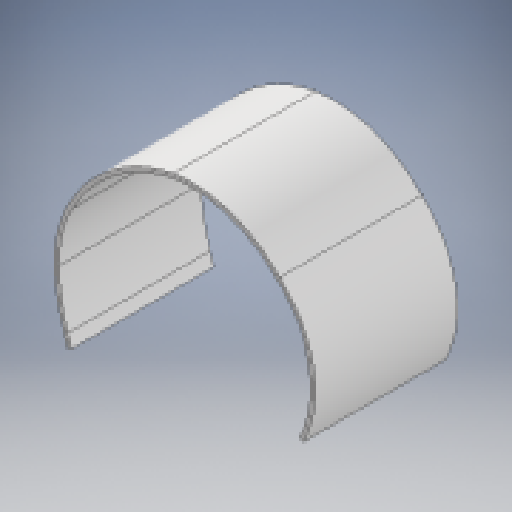
# Autodesk Inventor part: mount3
Saved by Autodesk Inventor 2025.2 (Build 292293000, 293)
## iProperties
Created: 2025-02-11
Part Number: mount3
Material: Generic
Document SubType Name: Modeling
Designer: Alex
Density: 1 g/cm^3
Appearance: Default
Author: Alex
Autodesk Inventor part; units mm, degrees
ref_plane "YZ Plane" through (0, 0, 0) normal (1, 0, 0) x (0, 1, 0)
ref_plane "XZ Plane" through (0, 0, 0) normal (0, 1, 0) x (-1, 0, 0)
ref_plane "XY Plane" through (0, 0, 0) normal (0, 0, 1) x (1, 0, 0)
sketch "Sketch1" plane through (0, 0, 0) normal (0, 0, 1) x (1, 0, 0)
  spline S0 degree 4 poles (-146.6472, 58.0401) (-151.4631, 48.7396) (-154.252, 35.0489) (-156.3713, 15.6625) (-155.4501, -11.3591) (-147.1073, -27.1547) (-140.0741, -39.9858) (-129.6609, -50.3249) (-121.6575, -59.5045) (-108.3024, -68.785) (-98.2709, -73.1981) (-84.1702, -79.7266) (-75.9561, -81.5933) (-64.5094, -82.4436) (-52.8851, -81.3854) (-36.0893, -77.2113) (-27.9896, -73.4594) (-12.8633, -65.2256) (-3.7509, -56.3713) (7.8984, -44.4028) (15.2147, -32.4708) (21.1011, -10.2225) (21.2051, 16.649) (15.9713, 25.1459) (12.5155, 32.2876) knots 0 0 0 0 0 0.111891 0.158364 0.204234 0.248308 0.289897 0.330614 0.370754 0.411053 0.44968 0.486304 0.522824 0.560101 0.5983 0.638491 0.679191 0.71966 0.761289 0.803726 0.849038 0.894451 1 1 1 1 1 construction
  arc A0 (-146.6314, -27.8645) -> (-75.5, -81.3478) centre (-54.4542, 20.6856) ccw construction
  arc A1 (-75.5, -81.3478) -> (-3.571, -56.0466) centre (-63.9052, 0.5835) ccw construction
  arc A2 (-155.7423, 8.5009) -> (-146.6314, -27.8645) centre (-64.0155, 12.158) ccw construction
  arc A3 (-146.6472, 58.0401) -> (-155.7423, 8.5009) centre (-41.1628, 13.0692) ccw construction
  arc A4 (-3.571, -56.0466) -> (18.787, -15.947) centre (-44.8542, -6.7459) ccw construction
  arc A5 (18.787, -15.947) -> (12.5155, 32.2876) centre (-51.5039, -0.5612) ccw construction
  arc A6 (-149.4068, 59.2166) -> (-149.2857, -29.2626) centre (-45.9699, 15.1186) ccw construction
  arc A7 (-149.2857, -29.2626) -> (-75.9204, -84.3182) centre (-62.5938, 9.8502) ccw construction
  arc A8 (-75.9204, -84.3182) -> (-1.3836, -58.0997) centre (-63.9052, 0.5835) ccw construction
  arc A9 (-1.3836, -58.0997) -> (15.1847, 33.6571) centre (-53.1101, -1.3853) ccw construction
  line L0 (-146.6472, 58.0401) -> (-149.4068, 59.2166) construction
  line L1 (-146.6314, -27.8645) -> (-149.2857, -29.2626) construction
  line L2 (-75.5, -81.3478) -> (-75.9204, -84.3182) construction
  line L3 (12.5155, 32.2876) -> (15.1847, 33.6571) construction
  line L4 (-3.571, -56.0466) -> (-1.3836, -58.0997) construction
  line L5 (-266.975, 160) -> (333.025, 160) construction
  line L6 (0, 160) -> (0, 0) construction
  arc A10 (-155.7423, 311.4991) -> (-146.6472, 261.9599) centre (-41.1628, 306.9308) ccw construction
  line L7 (-146.6472, 261.9599) -> (-149.4068, 260.7834) construction
  arc A11 (-149.2857, 349.2626) -> (-149.4068, 260.7834) centre (-45.9699, 304.8814) ccw construction
  spline S1 degree 4 poles (-146.6472, 261.9599) (-151.4631, 271.2604) (-154.252, 284.9511) (-156.3713, 304.3375) (-155.4501, 331.3591) (-147.1073, 347.1547) (-140.0741, 359.9858) (-129.6609, 370.3249) (-121.6575, 379.5045) (-108.3024, 388.785) (-98.2709, 393.1981) (-84.1702, 399.7266) (-75.9561, 401.5933) (-64.5094, 402.4436) (-52.8851, 401.3854) (-36.0893, 397.2113) (-27.9896, 393.4594) (-12.8633, 385.2256) (-3.7509, 376.3713) (7.8984, 364.4028) (15.2147, 352.4708) (21.1011, 330.2225) (21.2051, 303.351) (15.9713, 294.8541) (12.5155, 287.7124) knots 0 0 0 0 0 0.111891 0.158364 0.204234 0.248308 0.289897 0.330614 0.370754 0.411053 0.44968 0.486304 0.522824 0.560101 0.5983 0.638491 0.679191 0.71966 0.761289 0.803726 0.849038 0.894451 1 1 1 1 1 construction
  line L8 (-146.6314, 347.8645) -> (-149.2857, 349.2626) construction
  arc A12 (-75.5, 401.3478) -> (-146.6314, 347.8645) centre (-54.4542, 299.3144) ccw
  arc A13 (-75.9204, 404.3182) -> (-149.2857, 349.2626) centre (-62.5938, 310.1498) ccw construction
  line L9 (-3.571, 376.0466) -> (-1.3836, 378.0997) construction
  arc A14 (18.787, 335.947) -> (-3.571, 376.0466) centre (-44.8542, 326.7459) ccw
  line L10 (12.5155, 287.7124) -> (15.1847, 286.3429)
  arc A15 (12.5155, 287.7124) -> (18.787, 335.947) centre (-51.5039, 320.5612) ccw
  arc A16 (15.1847, 286.3429) -> (-1.3836, 378.0997) centre (-53.1101, 321.3853) ccw
  line L11 (-75.5, 401.3478) -> (-75.9204, 404.3182) construction
  arc A17 (-3.571, 376.0466) -> (-75.5, 401.3478) centre (-63.9052, 319.4165) ccw
  arc A18 (-1.3836, 378.0997) -> (-75.9204, 404.3182) centre (-63.9052, 319.4165) ccw construction
  line L12 (-154.6747, 292.7544) -> (-154.9494, 292.7201) construction
  arc A19 (-146.6314, 347.8645) -> (-154.9494, 292.7201) centre (-77.102, 309.1771) ccw construction
  arc A20 (-154.9494, 292.7201) -> (-148.0627, 261.3564) centre (-5.838, 309.0235) ccw construction
  arc A21 (-156.6572, 307.7541) -> (-151.3647, 272.6644) centre (-21.6788, 310.1684) ccw
  arc A22 (-151.3647, 272.6644) -> (-148.0627, 261.3564) centre (-5.838, 309.0235) ccw
  arc A23 (-146.6314, 347.8645) -> (-156.6572, 307.7541) centre (-77.102, 309.1771) ccw
  line L13 (-154.295, 328.4719) -> (-157.2055, 329.1994) construction
  line L14 (-151.3647, 272.6644) -> (-154.2753, 271.9372) construction
  line L15 (-148.0627, 261.3564) -> (-149.2046, 260.9737) construction
  arc A24 (-154.2753, 271.9372) -> (-150.9072, 260.4031) centre (-5.838, 309.0235) ccw
  line L16 (-148.0627, 261.3564) -> (-150.9072, 260.4031)
  line L17 (-156.6572, 307.7541) -> (-159.6572, 307.7541) construction
  arc A25 (-149.2857, 349.2626) -> (-157.2055, 329.1994) centre (-77.1444, 309.1907) ccw
  arc A26 (-157.2055, 329.1994) -> (-159.6572, 307.7541) centre (-77.1285, 309.1819) ccw
  line L18 (-155.169, 290.0346) -> (-158.1354, 289.5872) construction
  arc A27 (-159.6572, 307.7541) -> (-158.1354, 289.5872) centre (-21.7855, 310.1559) ccw
  arc A28 (-158.1354, 289.5872) -> (-154.2753, 271.9372) centre (-22.13, 310.0851) ccw
  line L19 (-153.9039, 339.4908) -> (-151.1134, 338.3893) construction
  line L20 (-159.1353, 318.5572) -> (-156.1548, 318.2165) construction
  line L21 (-159.1968, 298.6455) -> (-156.2073, 298.8959) construction
  line L22 (-156.4955, 280.6987) -> (-153.5647, 281.3397) construction
  line L23 (-152.7045, 266.1371) -> (-149.8248, 266.978) construction
  arc A29 (-75.9204, 404.3182) -> (-149.2857, 349.2626) centre (-54.4687, 299.3225) ccw
  line L24 (-117.0639, 382.5836) -> (-118.7912, 385.0365) construction
  arc A30 (-1.3836, 378.0997) -> (-75.9204, 404.3182) centre (-63.9052, 319.4165) ccw
  line L25 (-35.4522, 400.3059) -> (-36.4476, 397.4759) construction
  point P0 (-152, 43.3122)
  point P1 (-154.6747, 27.2456)
  point P2 (-153.5964, -11.5828)
  point P3 (-138.8691, -40.1727)
  point P4 (-129.9379, -50.283)
  point P5 (-120.8201, -59.3062)
  point P6 (-108.4988, -68.0622)
  point P7 (-96.8904, -73.8657)
  point P8 (-84.0513, -79.2561)
  point P9 (-65.5876, -82.0533)
  point P10 (-52.9328, -80.9408)
  point P11 (-37.3177, -77.1093)
  point P12 (-27.2436, -72.8759)
  point P13 (-14.2486, -65.2165)
  point P14 (6.8037, -44.6606)
  point P15 (14.0551, -32.7718)
  point P16 (19.9901, 7.1365)
  point P17 (16.9383, 22.5323)
  point P18 (0, 320)
  point P19 (-152, 276.6878)
  point P20 (-153.5964, 331.5828)
  point P21 (-138.8691, 360.1727)
  point P22 (-129.9379, 370.283)
  point P23 (-120.8201, 379.3062)
  point P24 (-108.4988, 388.0622)
  point P25 (-96.8904, 393.8657)
  point P26 (-84.0513, 399.2561)
  point P27 (-65.5876, 402.0533)
  point P28 (-52.9328, 400.9408)
  point P29 (-37.3177, 397.1093)
  point P30 (-27.2436, 392.8759)
  point P31 (-14.2486, 385.2165)
  point P32 (6.8037, 364.6606)
  point P33 (14.0551, 352.7718)
  point P34 (19.9901, 312.8635)
  point P35 (16.9383, 297.4677)
  point P36 (0, 320)
  dimension "d0" = 32.2876
  dimension "d1" = 12.5155
  dimension "d2" = 146.6472
  dimension "d3" = 58.0401
  dimension "d4" = 21.2257
  dimension "d5" = 24.6426
  dimension "d6" = 28.1888
  dimension "d7" = 35.6586
  dimension "d8" = 45.1759
  dimension "d9" = 56.1603
  dimension "d10" = 66.7549
  dimension "d11" = 77.8017
  dimension "d12" = 85.6648
  dimension "d13" = 96.7125
  dimension "d14" = 105.0451
  dimension "d15" = 110.9852
  dimension "d16" = 115.5255
  dimension "d17" = 121.8355
  dimension "d18" = 128.0798
  dimension "d19" = 134.591
  dimension "d20" = 139.3278
  dimension "d21" = 144.563
  dimension "d22" = 149.2554
  dimension "d23" = 158.0504
  dimension "d24" = 154.0325
  dimension "d25" = 157.056
  dimension "d26" = 155.9742
  dimension "d27" = 23.1148
  dimension "d28" = 15.6954
  dimension "d29" = 40.3471
  dimension "d30" = 26.2383
  dimension "d31" = 53.4492
  dimension "d32" = 67.4331
  dimension "d33" = 80.0452
  dimension "d34" = 92.9139
  dimension "d35" = 101.8898
  dimension "d36" = 114.3475
  dimension "d37" = 130.1838
  dimension "d38" = 135.2342
  dimension "d39" = 142.2055
  dimension "d40" = 148.8765
  dimension "d41" = 155.6989
  dimension "d42" = 160.5472
  dimension "d43" = 165.754
  dimension "d44" = 170.2579
  dimension "d45" = 175.7534
  dimension "d46" = 175.8185
  dimension "d47" = 175.7377
  dimension "d48" = 107.1872
  dimension "d49" = 172.4386
  dimension "d50" = 114.6706
  dimension "d51" = 104.1813
  dimension "d52" = 82.7477
  dimension "d53" = 64.3029
  dimension "d54" = 71.955
  dimension "d55" = 3
  dimension "d56" = 3
  dimension "d57" = 3
  dimension "d58" = 3
  dimension "d59" = 3
  dimension "d60" = 600
  dimension "d61" = 160
  dimension "d64" = 150
  dimension "d65" = 135
  constraints: 82 point on circle, 52 end point, 41 symmetric about line, 31 centre point, 19 line through centre, 2 coincident, 2 horizontal, 2 point on line, 2 tangent, 1 concentric, 1 perpendicular, 59 other
  measures "d0" vertical distance of L6.end L3.start
  measures "d1" horizontal distance of L6.end L3.start
  measures "d2" horizontal distance of L6.end L0.start
  measures "d3" vertical distance of L0.start L6.end
  measures "d4" distance of point (19.99, 7.136) L6.end
  measures "d5" distance of A4.end L6.end
  measures "d6" distance of point (16.938, 22.532) L6.end
  measures "d7" distance of point (14.055, -32.772) L6.end
  measures "d8" distance of point (6.804, -44.661) L6.end
  measures "d9" distance of L4.start L6.end
  measures "d10" distance of point (-14.249, -65.217) L6.end
  measures "d11" distance of point (-27.244, -72.876) L6.end
  measures "d12" distance of point (-37.318, -77.109) L6.end
  measures "d13" distance of point (-52.933, -80.941) L6.end
  measures "d14" distance of point (-65.588, -82.053) L6.end
  measures "d15" distance of L2.start L6.end
  measures "d16" distance of point (-84.051, -79.256) L6.end
  measures "d17" distance of point (-96.89, -73.866) L6.end
  measures "d18" distance of point (-108.499, -68.062) L6.end
  measures "d19" distance of point (-120.82, -59.306) L6.end
  measures "d20" distance of point (-129.938, -50.283) L6.end
  measures "d21" distance of point (-138.869, -40.173) L6.end
  measures "d22" distance of L1.start L6.end
  measures "d23" distance of point (-152, 43.312) L6.end
  measures "d24" distance of point (-153.596, -11.583) L6.end
  measures "d25" distance of point (-154.675, 27.246) L6.end
  measures "d26" distance of A3.end L6.end
  measures "d27" distance of point (19.99, 7.136) A4.end
  measures "d28" distance of point (19.99, 7.136) point (16.938, 22.532)
  measures "d29" distance of point (19.99, 7.136) point (14.055, -32.772)
  measures "d30" distance of point (19.99, 7.136) L3.start
  measures "d31" distance of point (19.99, 7.136) point (6.804, -44.661)
  measures "d32" distance of point (19.99, 7.136) L4.start
  measures "d33" distance of point (19.99, 7.136) point (-14.249, -65.217)
  measures "d34" distance of point (19.99, 7.136) point (-27.244, -72.876)
  measures "d35" distance of point (19.99, 7.136) point (-37.318, -77.109)
  measures "d36" distance of point (19.99, 7.136) point (-52.933, -80.941)
  measures "d37" distance of point (19.99, 7.136) L2.start
  measures "d38" distance of point (19.99, 7.136) point (-84.051, -79.256)
  measures "d39" distance of point (19.99, 7.136) point (-96.89, -73.866)
  measures "d40" distance of point (19.99, 7.136) point (-108.499, -68.062)
  measures "d41" distance of point (19.99, 7.136) point (-120.82, -59.306)
  measures "d42" distance of point (19.99, 7.136) point (-129.938, -50.283)
  measures "d43" distance of point (19.99, 7.136) point (-138.869, -40.173)
  measures "d44" distance of point (19.99, 7.136) L1.start
  measures "d45" distance of point (19.99, 7.136) point (-152, 43.312)
  measures "d46" distance of point (19.99, 7.136) point (-154.675, 27.246)
  measures "d47" distance of point (19.99, 7.136) A3.end
  measures "d48" distance of A4.end point (-65.588, -82.053)
  measures "d49" distance of A4.end point (-153.596, -11.583)
  measures "d50" radius of A3
  measures "d51" radius of A0
  measures "d52" radius of A1
  measures "d53" radius of A4
  measures "d54" radius of A5
  measures "d55" distance of L0.start L0.end
  measures "d56" distance of L1.start L1.end
  measures "d57" distance of L2.start L2.end
  measures "d58" distance of L3.start L3.end
  measures "d59" distance of L4.end L4.start
  measures "d60" distance of L5.start L5.end
  measures "d61" distance of L6.start L6.end
  measures "d64" radius of A20
  measures "d65" radius of A21
extrude "Extrusion1" add sketch "Sketch1" against normal blind 200
body "Solid1"
